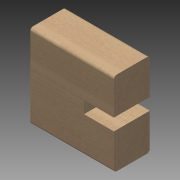
# Autodesk Inventor part: 2x4x3.5
Saved by Autodesk Inventor 2014 (Build 180170000, 170)
## iProperties
Created: 2013-10-13
Part Number: 2x4x3.5
Material: Ash
Document SubType Name: Modeling
Designer: david
Density: 0.641 g/cm^3
Appearance: Ash Door
Author: david
Autodesk Inventor part; units mm, degrees
ref_plane "YZ Plane" through (0, 0, 0) normal (1, 0, 0) x (0, 1, 0)
ref_plane "XZ Plane" through (0, 0, 0) normal (0, 1, 0) x (-1, 0, 0)
ref_plane "XY Plane" through (0, 0, 0) normal (0, 0, 1) x (1, 0, 0)
sketch "Sketch1" plane through (0, 0, 0) normal (1, 0, 0) x (0, 1, 0)
  line L0 (-3.7488, 0) -> (85.1512, 0)
  line L1 (85.1512, 0) -> (85.1512, 38.1)
  line L2 (85.1512, 38.1) -> (-3.7488, 38.1)
  line L3 (-3.7488, 38.1) -> (-3.7488, 0)
  point P0 (0, 0)
  dimension "d0" = 88.9
  dimension "d1" = 38.1
  constraints: 8 end point, 2 parallel, 1 horizontal, 1 perpendicular
  measures "d0" distance of L0.start L0.end
  measures "d1" distance of L2.end L0.start
extrude "Extrusion1" add sketch "Sketch1" along normal blind 88.9
fillet "Fillet1" radius 3.175 4 edges at (44.45, 85.1512, 38.1) (44.45, 85.1512, 0) (44.45, -3.7488, 0) (44.45, -3.7488, 38.1)
sketch "Sketch2" plane through (88.9, 0, 0) normal (1, 0, 0) x (0, 0, -1)
  line L0 (-34.925, -3.7488) -> (-3.175, -3.7488) projected
  line L1 (0, -0.5738) -> (0, 81.9762) projected
  line L2 (-3.175, 85.1512) -> (-34.925, 85.1512) projected
  line L3 (-38.1, 81.9762) -> (-38.1, -0.5738) projected
  line L4 (-38.1, 47.0512) -> (0, 47.0512)
  line L5 (0, 47.0512) -> (0, 34.3512)
  line L6 (0, 34.3512) -> (-38.1, 34.3512)
  line L7 (-38.1, 34.3512) -> (-38.1, 47.0512)
  point P0 (0, 0)
  dimension "d5" = 38.1
  dimension "d6" = 38.1
  constraints: 8 end point, 2 parallel, 2 point on line, 1 horizontal, 1 perpendicular
  measures "d5" distance between parallel lines of L2 L4
  measures "d6" distance between parallel lines of L0 L6
extrude "Extrusion2" cut sketch "Sketch2" against normal blind 31.75
body "Solid1"
